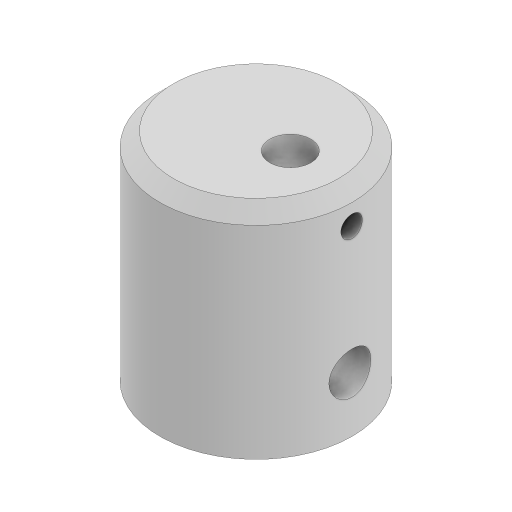
# Autodesk Inventor part: Spigot
Saved by Autodesk Inventor 2023.2 (Build 272271030, 271C)
## iProperties
Created: 2023-09-12
Part Number: Spigot
Material: Generic
Document SubType Name: Modeling
Designer: User
Mass: 15.0142 g
Surface Area: 52.3532 cm^2
Volume: 15.0142 cm^3
Density: 1 g/cm^3
Appearance: Default
Author: User
Autodesk Inventor part; units mm, degrees
ref_plane "YZ Plane" through (0, 0, 0) normal (1, 0, 0) x (0, 1, 0)
ref_plane "XZ Plane" through (0, 0, 0) normal (0, 1, 0) x (-1, 0, 0)
ref_plane "XY Plane" through (0, 0, 0) normal (0, 0, 1) x (1, 0, 0)
sketch "Sketch1" plane through (0, 0, 0) normal (0, 0, 1) x (1, 0, 0)
  line L0 (0, 0) -> (14, 0)
  line L1 (14, 0) -> (14, 31.5)
  line L2 (14, 31.5) -> (0, 31.5)
  line L3 (0, 31.5) -> (0, 0)
  dimension "d1" = 31.5
  dimension "d31" = 28
  constraints: 8 end point, 2 parallel, 1 horizontal, 1 perpendicular
  measures "d1" distance of L0.end L1.end
  measures "d31" diameter of L1 L3
revolve "Revolution1" add sketch "Sketch1" angle 360 about axis through (0, 31.5, 0) along (0, -1, 0)
chamfer "Chamfer1" distance 2 angle 45 1 edges at (-14, 31.5, 0)
sketch "Sketch2" plane through (0, 0, 0) normal (0, 0, 1) x (1, 0, 0)
  line L0 (-14, 29.5) -> (-14, 0) projected
  line L1 (14, 29.5) -> (14, 0) projected
  line L2 (-14, 26.5) -> (14, 26.5)
  line L3 (-14, 8) -> (14, 8)
  line L4 (-14, 27.5) -> (14, 28.06)
  line L5 (-14, 10.5) -> (14, 11.06)
  line L6 (-12, 31.5) -> (12, 31.5) projected
  line L7 (-14, 0) -> (14, 0) projected
  line L8 (-14, 27.5) -> (-14, 26.5)
  line L9 (14, 28.06) -> (14, 26.5)
  line L10 (14, 11.06) -> (14, 8)
  line L11 (-14, 10.5) -> (-14, 8)
  point P0 (0, 0)
  dimension "d6" = 1
  dimension "d8" = 1.56
  dimension "d9" = 2.5
  dimension "d10" = 3.06
  dimension "d12" = 8
  dimension "d13" = 5
  constraints: 16 end point, 8 point on line, 4 collinear, 2 perpendicular
  measures "d6" distance of L4.start L2.start
  measures "d8" distance of L2.end L4.end
  measures "d9" distance of L3.start L5.start
  measures "d10" distance of L3.end L5.end
  measures "d12" distance of L1.end L3.end
  measures "d13" vertical distance of L6.end L2.end
revolve "Revolution2" cut sketch "Sketch2" angle 360 about axis through (-14, 26.5, 0) along (1, 0, 0) contours L4 L1 L2 L0
revolve "Revolution3" cut sketch "Sketch2" angle 360 about axis through (-14, 8, 0) along (1, 0, 0) contours L5 L1 L3 L0
sketch "Sketch3" plane through (0, 0, 0) normal (0, -1, 0) x (1, 0, 0)
  circle A0 centre (0, 0) radius 14 projected
hole "Hole1" at (0, 0, 0) direction (0, 1, 0) diameter 15 depth 18 tip angle 118
sketch "Sketch4" plane through (0, 31.5, 0) normal (0, 1, 0) x (1, 0, 0)
  circle A0 centre (0, 0) radius 12 projected
  point P0 (5, 0)
  dimension "d23" = 5
  constraints: 1 horizontal alignment
  measures "d23" distance of point (5, 0) A0.centre
hole "Hole2" at (5, 31.5, 0) direction (0, -1, 0) diameter 6 depth 12 tip angle 118
sketch "Sketch5" plane through (0, 0, 0) normal (0, 0, 1) x (1, 0, 0)
  point P0 (0, 0)
equation "\"d8\" = d6 + 0.02 * d0"
equation "\"d10\" = d9 + 0.02 * d0"
equation "\"d0\" = 28"
body "Solid1"
